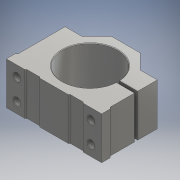
# Autodesk Inventor part: SMK52
Saved by Autodesk Inventor 2016 (Build 200138000, 138)
## iProperties
Created: 2016-10-22
Part Number: SMK52
Material: Типовые
Document SubType Name: Modeling
Designer: skhalipa
Density: 1 g/cm^3
Appearance: Анодированный — светло-серый
Author: skhalipa
Autodesk Inventor part; units mm, degrees
ref_plane "YZ Plane" through (0, 0, 0) normal (1, 0, 0) x (0, 1, 0)
ref_plane "XZ Plane" through (0, 0, 0) normal (0, 1, 0) x (-1, 0, 0)
ref_plane "XY Plane" through (0, 0, 0) normal (0, 0, 1) x (1, 0, 0)
sketch "Эскиз1" plane through (0, 0, 0) normal (0, 0, 1) x (1, 0, 0)
  line L0 (-45, 34) -> (45, 34)
  line L1 (45, 34) -> (45, -34)
  line L2 (45, -34) -> (-45, -34)
  line L3 (-45, -34) -> (-45, 34)
  point P0 (0, 0)
  point P1 (-45, 0)
  point P2 (0, 34)
  dimension "d0" = 90
  dimension "d1" = 68
  constraints: 8 end point, 2 midpoint, 2 parallel, 1 horizontal, 1 horizontal alignment, 1 perpendicular, 1 vertical alignment
  measures "d0" distance of L0.start L0.end
  measures "d1" distance of L2.end L0.start
extrude "Выдавливание1" add sketch "Эскиз1" against normal blind 40
sketch "Эскиз2" plane through (0, 0, 0) normal (0, 0, 1) x (1, 0, 0)
  line L0 (-45, -34) -> (-45, 34) projected
  line L1 (-45, 20) -> (-27.5, 20)
  line L2 (-27.5, 20) -> (-13.5, 34)
  line L3 (-13.5, 34) -> (13.5, 34)
  line L4 (-45, 34) -> (45, 34) projected
  line L5 (13.5, 34) -> (27.5, 20)
  line L6 (27.5, 20) -> (45, 20)
  line L7 (45, 34) -> (45, -34) projected
  line L8 (45, -34) -> (-45, -34) projected
  point P0 (0, 0)
  dimension "d4" = 27
  dimension "d5" = 55
  dimension "d6" = 17.5
  dimension "d7" = 14
  dimension "d8" = 54
  dimension "d9" = 135
  constraints: 10 end point, 5 point on line, 1 horizontal
  measures "d4" distance of L3.end L2.end
  measures "d5" distance of L5.end L1.end
  measures "d6" distance of L1.start L1.end
  measures "d7" horizontal distance of L2.end L1.end
  measures "d8" distance between parallel lines of L8 L1
  measures "d9" angle of L2 L1
extrude "Выдавливание2" cut sketch "Эскиз2" against normal blind 40 contours L0 L4 L2 L1 | L6 L5 L4 L7
sketch "Эскиз3" plane through (0, 0, 0) normal (0, 0, 1) x (1, 0, 0)
  line L0 (-45, 20) -> (-27.5, 20) projected
  line L1 (-43.5, 20) -> (-43.5, -24.5)
  line L2 (-43.5, -24.5) -> (-45, -26)
  line L3 (-45, -34) -> (-45, 20) projected
  line L4 (45, -34) -> (-45, -34) projected
  point P0 (0, 0)
  dimension "d12" = 1.5
  dimension "d13" = 1.5
  dimension "d14" = 8
  constraints: 4 end point, 2 point on line, 1 vertical
  measures "d12" distance between parallel lines of L1 L3
  measures "d13" horizontal distance of L2.end L1.end
  measures "d14" distance from line of L2.end L4
extrude "Выдавливание3" cut sketch "Эскиз3" against normal blind 40
sketch "Эскиз5" plane through (0, 0, 0) normal (0, 0, 1) x (1, 0, 0)
  line L0 (27.5, 20) -> (45, 20) projected
  line L1 (43.5, 20) -> (43.5, -24.5)
  line L2 (43.5, -24.5) -> (45, -26)
  line L3 (45, 20) -> (45, -34) projected
  point P0 (0, 0)
  point P1 (-43.5, -24.5)
  point P2 (-45, -26)
  dimension "d21" = 1.5
  constraints: 4 end point, 3 horizontal alignment, 2 point on line, 1 vertical
  measures "d21" distance between parallel lines of L3 L1
extrude "Выдавливание4" cut sketch "Эскиз5" against normal blind 40
sketch "Эскиз6" plane through (0, 0, 0) normal (0, 0, 1) x (1, 0, 0)
  circle A0 centre (0, 0) radius 26
  line L0 (25.9567, 1.5) -> (43.5, 1.5)
  line L1 (43.5, 20) -> (43.5, -24.5) projected
  line L2 (25.9567, -1.5) -> (43.5, -1.5)
  line L3 (45, -34) -> (-45, -34) projected
  point P0 (0, -26)
  dimension "d24" = 52
  dimension "d25" = 8
  dimension "d26" = 3
  dimension "d27" = 1.5
  constraints: 4 end point, 3 point on circle, 2 point on line, 1 centre point, 1 coincident, 1 horizontal, 1 parallel
  measures "d24" diameter of A0
  measures "d25" distance from line of L3 point (0, -26)
  measures "d26" distance between parallel lines of L0 L2
  measures "d27" distance from line of point (0, 0) L2
extrude "Выдавливание5" cut sketch "Эскиз6" against normal blind 40
sketch "Эскиз7" plane through (-45, -34, 0) normal (0, -1, 0) x (1, 0, 0)
  line L0 (90, 0) -> (0, 0) projected
  line L1 (0, 0) -> (0, -40) projected
  point P0 (45, 0)
  point P1 (80, -30)
  point P2 (80, -10)
  point P3 (10, -10)
  point P4 (10, -30)
  dimension "d30" = 20
  dimension "d31" = 70
  dimension "d32" = 10
  dimension "d33" = 10
  constraints: 2 horizontal alignment, 2 vertical alignment
  measures "d30" distance of point (80, -10) point (80, -30)
  measures "d31" distance of point (10, -10) point (80, -10)
  measures "d32" distance from line of L0 point (10, -10)
  measures "d33" distance from line of L1 point (10, -10)
hole "Отверстие1" at (35, -34, -30) at (35, -34, -10) at (-35, -34, -10) at (-35, -34, -30) direction (0, 1, 0) diameter 6.5 end through all
chamfer "Фаска1" distance 0.5 angle 45 10 edges at (35, 20, -26.75) (35, 20, -6.75) (-35, 20, -26.75) (-35, 20, -6.75) (-26, 0, -40) (-26, 0, 0) (35, -34, -26.75) (-35, -34, -26.75) (35, -34, -6.75) (-35, -34, -6.75)
sketch "Эскиз8" plane through (0, 0, 0) normal (0, 0, 1) x (1, 0, 0)
  line L0 (45, -34) -> (-45, -34) projected
  line L1 (-27.5, -34) -> (-26.5, -33)
  line L2 (-26.5, -33) -> (-14.5, -33)
  line L3 (-14.5, -33) -> (-13.5, -34)
  line L4 (13.5, -34) -> (14.5, -33)
  line L5 (14.5, -33) -> (26.5, -33)
  line L6 (26.5, -33) -> (27.5, -34)
  point P0 (0, 0)
  point P1 (-27.5, 20)
  point P2 (-13.5, 34)
  point P3 (13.5, 34)
  point P4 (27.5, 20)
  dimension "d44" = 1
  dimension "d45" = 45
  dimension "d46" = 45
  dimension "d47" = 45
  constraints: 12 end point, 6 point on line, 4 vertical alignment, 2 parallel
  measures "d44" distance between parallel lines of L0 L2
  measures "d45" angle of L0 L1
  measures "d46" angle of L0 L3
  measures "d47" angle of L4 L0
extrude "Выдавливание6" cut sketch "Эскиз8" against normal blind 40
